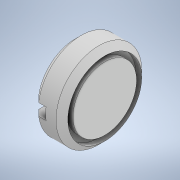
# Autodesk Inventor part: 711118
Saved by Autodesk Inventor 2022 (Build 260153000, 153)
## iProperties
Created: 2021-10-21
Part Number: 711118
Material: Типовые
Document SubType Name: Modeling
Designer: RaNSiD
Density: 1 g/cm^3
Appearance: По умолчанию
Mass: 21.1908 g
Surface Area: 62.2851 cm^2
Volume: 21.1908 cm^3
Author: RaNSiD
Autodesk Inventor part; units mm, degrees
ref_plane "YZ Plane" through (0, 0, 0) normal (1, 0, 0) x (0, 1, 0)
ref_plane "XZ Plane" through (0, 0, 0) normal (0, 1, 0) x (-1, 0, 0)
ref_plane "XY Plane" through (0, 0, 0) normal (0, 0, 1) x (1, 0, 0)
sketch "Эскиз5" plane through (0, 0, 0) normal (0, 0, 1) x (1, 0, 0)
  line L0 (0, 0) -> (20, 0)
  line L1 (20, 0) -> (20, 25)
  line L2 (16, 29) -> (4, 29)
  line L3 (0, 25) -> (0, 0)
  line L4 (4, 29) -> (0, 25)
  line L5 (16, 29) -> (20, 25)
  point P0 (20, 29)
  point P1 (0, 29)
  dimension "d23" = 20
  dimension "d24" = 29
  dimension "d25" = 4
  dimension "d26" = 4
  dimension "d27" = 4
  dimension "d28" = 4
  constraints: 12 end point, 4 point on line, 2 parallel, 1 horizontal, 1 perpendicular
  measures "d23" distance of point (0, 29) point (20, 29)
  measures "d24" distance of point (20, 29) L0.end
  measures "d25" distance of L2.end point (0, 29)
  measures "d26" distance of L3.start point (0, 29)
  measures "d27" distance of L2.start point (20, 29)
  measures "d28" distance of L1.end point (20, 29)
revolve "Вращение3" add sketch "Эскиз5" angle 360 about axis through (0, 0, 0) along (1, 0, 0)
sketch "Эскиз6" plane through (0, 0, 0) normal (0, 0, 1) x (1, 0, 0)
  line L0 (0, -25) -> (0, 25) construction
  line L1 (0, 4) -> (9, 4)
  line L2 (9, 4) -> (9, -4)
  line L3 (9, -4) -> (0, -4)
  line L4 (0, -4) -> (0, 4)
  point P0 (0, 0)
  point P1 (0, 0)
  point P2 (0, 0)
  dimension "d30" = 9
  dimension "d31" = 8
  constraints: 8 end point, 2 midpoint, 2 parallel, 1 coincident, 1 horizontal, 1 perpendicular, 1 point on line
  measures "d30" distance of L2.end L3.end
  measures "d31" distance of L1.end L2.end
extrude "Выдавливание2" cut sketch "Эскиз6" along normal through all both and the other way through all
sketch "Эскиз7" plane through (0, 0, 0) normal (-1, 0, 0) x (0, 0, 1)
  line L0 (0, 0) -> (0, 20) construction
  dimension "d34" = 20
  constraints: 2 end point, 1 coincident, 1 vertical
  measures "d34" distance of L0.start L0.end
hole "Отверстие2" at (0, 20, 0) direction (1, 0, 0) diameter 4 depth 4 tip angle 118
sketch "Эскиз8" plane through (0, 0, 0) normal (0, 0, 1) x (1, 0, 0)
  line L0 (20, -25) -> (20, 25) construction
  line L1 (20, 25) -> (16, 25)
  line L2 (16, 25) -> (16, 21.5)
  line L3 (16, 21.5) -> (20, 21.5)
  line L4 (20, 21.5) -> (20, 25)
  line L5 (0, 0) -> (20, 0)
  dimension "d42" = 4
  dimension "d43" = 3.5
  constraints: 10 end point, 2 parallel, 1 horizontal, 1 midpoint, 1 perpendicular
  measures "d42" distance of L3.end L2.end
  measures "d43" distance of L2.end L1.end
revolve "Вращение4" cut sketch "Эскиз8" angle 360 about axis through (0, 0, 0) along (1, 0, 0)
equation "\"d26\" = d25"
equation "\"d27\" = d25"
equation "\"d28\" = d27"
